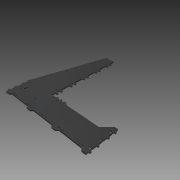
# Autodesk Inventor part: brace_right
Saved by Autodesk Inventor 2014 (Build 180170000, 170)
## iProperties
Created: 2013-12-03
Part Number: brace_right
Material: Generic
Document SubType Name: Modeling
Designer: buben
Density: 1 g/cm^3
Appearance: Anodized - Dark Gray
Author: buben
Subject: Laser Cutted
Autodesk Inventor part; units mm, degrees
ref_plane "YZ Plane" through (0, 0, 0) normal (1, 0, 0) x (0, 1, 0)
ref_plane "XZ Plane" through (0, 0, 0) normal (0, 1, 0) x (-1, 0, 0)
ref_plane "XY Plane" through (0, 0, 0) normal (0, 0, 1) x (1, 0, 0)
sketch "Sketch1" plane through (0, 0, 0) normal (0, 0, 1) x (1, 0, 0)
  line L0 (0, 0) -> (489, 0)
  line L1 (489, 0) -> (489, 150)
  line L2 (0, 0) -> (0, 120)
  line L3 (0, 120) -> (106.25, 518.5)
  line L4 (106.25, 518.5) -> (156.25, 518.5)
  line L5 (156.25, 518.5) -> (156.25, 113.5)
  line L6 (489, 150) -> (474, 150)
  line L7 (474, 150) -> (434, 110)
  line L8 (434, 110) -> (253.25, 110)
  line L9 (253.25, 110) -> (243.25, 120)
  line L10 (243.25, 120) -> (233.25, 120)
  line L11 (233.25, 120) -> (233.25, 113.5)
  line L12 (233.25, 113.5) -> (156.25, 113.5)
  point P0 (244.5, 0)
  dimension "d0" = 489
  dimension "d2" = 120
  dimension "d3" = 45
  dimension "d5" = 6.5
  dimension "d6" = 77
  dimension "d7" = 15
  dimension "d8" = 10
  dimension "d9" = 50
  dimension "d10" = 518.5
  dimension "d13" = 10
  dimension "d261" = 156.25
  dimension "d289" = 150
  dimension "d290" = 40
  constraints: 26 end point, 7 perpendicular, 3 parallel, 1 horizontal, 1 midpoint
  measures "d0" distance of L0.start L0.end
  measures "d2" distance of L0.start L2.end
  measures "d3" angle of L6 L7
  measures "d5" distance of L10.end L11.end
  measures "d6" distance of L11.end L5.end
  measures "d7" distance of L1.end L6.end
  measures "d8" distance of L9.end L10.end
  measures "d9" distance of L3.end L4.end
  measures "d10" distance between parallel lines of L0 L4
  measures "d13" distance between parallel lines of L8 L10
  measures "d261" distance between parallel lines of L2 L5
  measures "d289" distance of L0.end L1.end
  measures "d290" distance between parallel lines of L6 L8
extrude "Extrusion1" add sketch "Sketch1" along normal blind 6.5
sketch "Sketch20" plane through (0, 0, 6.5) normal (0, 0, 1) x (1, 0, 0)
  line L0 (0, 0) -> (489, 0) projected
  line L1 (0, 120) -> (0, 0) projected
  line L2 (16.3, 20.75) -> (16.3, 16.25)
  line L3 (0, 16.25) -> (0, 20.75)
  line L4 (5, 23.25) -> (12.3, 23.25)
  line L5 (12.3, 13.75) -> (5, 13.75)
  line L6 (0, 20.75) -> (5, 20.75)
  line L7 (12.3, 20.75) -> (16.3, 20.75)
  line L8 (16.3, 16.25) -> (12.3, 16.25)
  line L9 (5, 16.25) -> (0, 16.25)
  line L10 (5, 13.75) -> (5, 16.25)
  line L11 (5, 20.75) -> (5, 23.25)
  line L12 (12.3, 23.25) -> (12.3, 20.75)
  line L13 (12.3, 16.25) -> (12.3, 13.75)
  line L14 (16.3, 59.75) -> (16.3, 55.25)
  line L15 (0, 55.25) -> (0, 59.75)
  line L16 (5, 62.25) -> (12.3, 62.25)
  line L17 (12.3, 52.75) -> (5, 52.75)
  line L18 (0, 59.75) -> (5, 59.75)
  line L19 (12.3, 59.75) -> (16.3, 59.75)
  line L20 (16.3, 55.25) -> (12.3, 55.25)
  line L21 (5, 55.25) -> (0, 55.25)
  line L22 (5, 52.75) -> (5, 55.25)
  line L23 (5, 59.75) -> (5, 62.25)
  line L24 (12.3, 62.25) -> (12.3, 59.75)
  line L25 (12.3, 55.25) -> (12.3, 52.75)
  line L26 (16.3, 98.75) -> (16.3, 94.25)
  line L27 (0, 94.25) -> (0, 98.75)
  line L28 (5, 101.25) -> (12.3, 101.25)
  line L29 (12.3, 91.75) -> (5, 91.75)
  line L30 (0, 98.75) -> (5, 98.75)
  line L31 (12.3, 98.75) -> (16.3, 98.75)
  line L32 (16.3, 94.25) -> (12.3, 94.25)
  line L33 (5, 94.25) -> (0, 94.25)
  line L34 (5, 91.75) -> (5, 94.25)
  line L35 (5, 98.75) -> (5, 101.25)
  line L36 (12.3, 101.25) -> (12.3, 98.75)
  line L37 (12.3, 94.25) -> (12.3, 91.75)
  point P0 (16.3, 18.5)
  point P1 (16.3, 57.5)
  point P2 (16.3, 96.5)
  dimension "d291" = 4.5
  dimension "d292" = 5
  dimension "d293" = 4
  dimension "d294" = 7.3
  dimension "d295" = 2.5
  dimension "d296" = 18.5
  dimension "d299" = 39
  constraints: 72 end point, 10 parallel, 6 collinear, 4 perpendicular, 3 horizontal, 1 midpoint, 1 vertical, 50 other
  measures "d291" distance of L2.start L2.end
  measures "d292" distance of L9.start L3.start
  measures "d293" distance of L2.end L8.end
  measures "d294" distance of L5.start L5.end
  measures "d295" distance of L5.end L9.start
  measures "d296" distance from line of L0 point (16.3, 18.5)
  measures "d299" distance of L2.start L19.end
extrude "Extrusion21" cut sketch "Sketch20" against normal through all
sketch "Sketch21" plane through (0, 0, 6.5) normal (0, 0, 1) x (1, 0, 0)
  line L0 (0, 55.25) -> (0, 20.75) projected
  line L1 (16.3, 20.75) -> (16.3, 16.25) projected
  line L2 (0, 16.25) -> (0, 0) projected
  line L3 (0, 120) -> (0, 98.75) projected
  line L4 (16.3, 98.75) -> (16.3, 94.25) projected
  line L5 (0, 94.25) -> (0, 59.75) projected
  line L6 (0, 112) -> (-4.5, 112)
  line L7 (-6.5, 110) -> (-6.5, 106)
  line L8 (-4.5, 104) -> (0, 104)
  line L9 (0, 104) -> (0, 112)
  line L10 (0, 81) -> (-4.5, 81)
  line L11 (-6.5, 79) -> (-6.5, 75)
  line L12 (-4.5, 73) -> (0, 73)
  line L13 (0, 73) -> (0, 81)
  line L14 (0, 42) -> (-4.5, 42)
  line L15 (-6.5, 40) -> (-6.5, 36)
  line L16 (-4.5, 34) -> (0, 34)
  line L17 (0, 34) -> (0, 42)
  line L18 (0, 11) -> (-4.5, 11)
  line L19 (-6.5, 9) -> (-6.5, 5)
  line L20 (-4.5, 3) -> (0, 3)
  line L21 (0, 3) -> (0, 11)
  arc A0 (-6.5, 5) -> (-4.5, 3) centre (-4.5, 5) ccw
  arc A1 (-4.5, 11) -> (-6.5, 9) centre (-4.5, 9) ccw
  arc A2 (-6.5, 36) -> (-4.5, 34) centre (-4.5, 36) ccw
  arc A3 (-4.5, 42) -> (-6.5, 40) centre (-4.5, 40) ccw
  arc A4 (-6.5, 75) -> (-4.5, 73) centre (-4.5, 75) ccw
  arc A5 (-4.5, 81) -> (-6.5, 79) centre (-4.5, 79) ccw
  arc A6 (-6.5, 106) -> (-4.5, 104) centre (-4.5, 106) ccw
  arc A7 (-4.5, 112) -> (-6.5, 110) centre (-4.5, 110) ccw
  point P0 (16.3, 96.5)
  point P1 (16.3, 18.5)
  point P2 (-6.5, 38)
  point P3 (0, 38)
  point P4 (-6.5, 77)
  point P5 (0, 77)
  dimension "d306" = 2
  dimension "d307" = 8
  dimension "d308" = 8
  dimension "d309" = 8
  dimension "d310" = 8
  dimension "d311" = 6.5
  dimension "d312" = 7.5
  dimension "d313" = 7.5
  constraints: 32 end point, 16 point on circle, 16 tangent, 8 centre point, 8 parallel, 7 equal radius, 6 midpoint, 4 horizontal, 4 perpendicular, 4 point on line, 3 collinear, 2 horizontal alignment
  measures "d306" radius of A0
  measures "d307" distance between parallel lines of L20 L18
  measures "d308" distance between parallel lines of L14 L16
  measures "d309" distance between parallel lines of L10 L12
  measures "d310" distance between parallel lines of L6 L8
  measures "d311" distance between parallel lines of L2 L19
  measures "d312" distance from line of L18 point (16.3, 18.5)
  measures "d313" distance from line of L8 point (16.3, 96.5)
extrude "Extrusion22" add sketch "Sketch21" against normal blind 6.5
sketch "Sketch22" plane through (0, 0, 6.5) normal (0, 0, 1) x (1, 0, 0)
  line L0 (233.25, 120) -> (233.25, 113.5) projected
  line L1 (233.25, 113.5) -> (156.25, 113.5) projected
  line L2 (201.5, 113.5) -> (206, 113.5)
  line L3 (206, 97.2) -> (201.5, 97.2)
  line L4 (208.5, 108.5) -> (208.5, 101.2)
  line L5 (199, 101.2) -> (199, 108.5)
  line L6 (206, 113.5) -> (206, 108.5)
  line L7 (206, 101.2) -> (206, 97.2)
  line L8 (201.5, 97.2) -> (201.5, 101.2)
  line L9 (201.5, 108.5) -> (201.5, 113.5)
  line L10 (199, 108.5) -> (201.5, 108.5)
  line L11 (206, 108.5) -> (208.5, 108.5)
  line L12 (208.5, 101.2) -> (206, 101.2)
  line L13 (201.5, 101.2) -> (199, 101.2)
  point P0 (203.75, 97.2)
  dimension "d316" = 4.5
  dimension "d317" = 5
  dimension "d318" = 7.3
  dimension "d319" = 4
  dimension "d320" = 2.5
  dimension "d321" = 29.5
  constraints: 24 end point, 10 parallel, 6 collinear, 4 perpendicular, 3 horizontal, 1 midpoint
  measures "d316" distance of L3.start L3.end
  measures "d317" distance of L2.end L6.end
  measures "d318" distance of L4.start L4.end
  measures "d319" distance of L7.start L3.start
  measures "d320" distance of L8.end L5.start
  measures "d321" distance from line of L0 point (203.75, 97.2)
extrude "Extrusion23" cut sketch "Sketch22" against normal through all
sketch "Sketch23" plane through (0, 0, 6.5) normal (0, 0, 1) x (1, 0, 0)
  line L0 (206, 97.2) -> (201.5, 97.2) projected
  line L1 (201.5, 113.5) -> (156.25, 113.5) projected
  line L2 (243.25, 120) -> (233.25, 120) projected
  line L3 (233.25, 113.5) -> (206, 113.5) projected
  line L4 (196.25, 113.5) -> (188.25, 113.5)
  line L5 (188.25, 113.5) -> (188.25, 118)
  line L6 (190.25, 120) -> (194.25, 120)
  line L7 (196.25, 118) -> (196.25, 113.5)
  line L8 (211.25, 113.5) -> (219.25, 113.5)
  line L9 (219.25, 113.5) -> (219.25, 118)
  line L10 (217.25, 120) -> (213.25, 120)
  line L11 (211.25, 118) -> (211.25, 113.5)
  arc A0 (190.25, 120) -> (188.25, 118) centre (190.25, 118) ccw
  arc A1 (196.25, 118) -> (194.25, 120) centre (194.25, 118) ccw
  arc A2 (213.25, 120) -> (211.25, 118) centre (213.25, 118) ccw
  arc A3 (219.25, 118) -> (217.25, 120) centre (217.25, 118) ccw
  point P0 (203.75, 97.2)
  dimension "d324" = 2
  dimension "d325" = 8
  dimension "d326" = 8
  dimension "d327" = 15
  dimension "d328" = 7.5
  constraints: 16 end point, 8 point on circle, 8 tangent, 4 centre point, 4 parallel, 3 equal radius, 2 collinear, 2 horizontal, 2 perpendicular, 2 point on line, 1 midpoint
  measures "d324" radius of A0
  measures "d325" distance between parallel lines of L7 L5
  measures "d326" distance between parallel lines of L9 L11
  measures "d327" distance between parallel lines of L11 L7
  measures "d328" distance from line of point (203.75, 97.2) L7
extrude "Extrusion24" add sketch "Sketch23" against normal blind 6.5
sketch "Sketch24" plane through (0, 0, 6.5) normal (0, 0, 1) x (1, 0, 0)
  line L0 (0, 3) -> (0, 0) projected
  line L1 (489, 0) -> (489, 150) projected
  line L2 (30, 9.5) -> (38, 9.5)
  line L3 (38, 9.5) -> (38, 3)
  line L4 (38, 3) -> (30, 3)
  line L5 (30, 3) -> (30, 9.5)
  line L6 (53, 9.5) -> (61, 9.5)
  line L7 (61, 9.5) -> (61, 3)
  line L8 (61, 3) -> (53, 3)
  line L9 (53, 3) -> (53, 9.5)
  circle A0 centre (45.5, 6.25) radius 2.25
  line L10 (129.5, 9.5) -> (137.5, 9.5)
  line L11 (137.5, 9.5) -> (137.5, 3)
  line L12 (137.5, 3) -> (129.5, 3)
  line L13 (129.5, 3) -> (129.5, 9.5)
  line L14 (152.5, 9.5) -> (160.5, 9.5)
  line L15 (160.5, 9.5) -> (160.5, 3)
  line L16 (160.5, 3) -> (152.5, 3)
  line L17 (152.5, 3) -> (152.5, 9.5)
  circle A1 centre (145, 6.25) radius 2.25
  line L18 (229, 9.5) -> (237, 9.5)
  line L19 (237, 9.5) -> (237, 3)
  line L20 (237, 3) -> (229, 3)
  line L21 (229, 3) -> (229, 9.5)
  line L22 (252, 9.5) -> (260, 9.5)
  line L23 (260, 9.5) -> (260, 3)
  line L24 (260, 3) -> (252, 3)
  line L25 (252, 3) -> (252, 9.5)
  circle A2 centre (244.5, 6.25) radius 2.25
  line L26 (328.5, 9.5) -> (336.5, 9.5)
  line L27 (336.5, 9.5) -> (336.5, 3)
  line L28 (336.5, 3) -> (328.5, 3)
  line L29 (328.5, 3) -> (328.5, 9.5)
  line L30 (351.5, 9.5) -> (359.5, 9.5)
  line L31 (359.5, 9.5) -> (359.5, 3)
  line L32 (359.5, 3) -> (351.5, 3)
  line L33 (351.5, 3) -> (351.5, 9.5)
  circle A3 centre (344, 6.25) radius 2.25
  line L34 (428, 9.5) -> (436, 9.5)
  line L35 (436, 9.5) -> (436, 3)
  line L36 (436, 3) -> (428, 3)
  line L37 (428, 3) -> (428, 9.5)
  line L38 (451, 9.5) -> (459, 9.5)
  line L39 (459, 9.5) -> (459, 3)
  line L40 (459, 3) -> (451, 3)
  line L41 (451, 3) -> (451, 9.5)
  circle A4 centre (443.5, 6.25) radius 2.25
  line L42 (61, 6.25) -> (129.5, 6.25) construction
  line L43 (160.5, 6.25) -> (229, 6.25) construction
  line L44 (260, 6.25) -> (328.5, 6.25) construction
  line L45 (359.5, 6.25) -> (428, 6.25) construction
  line L46 (0, 0) -> (489, 0) projected
  point P0 (38, 6.25)
  point P1 (137.5, 6.25)
  point P2 (237, 6.25)
  point P3 (336.5, 6.25)
  point P4 (436, 6.25)
  dimension "d331" = 8
  dimension "d332" = 6.5
  dimension "d333" = 15
  dimension "d334" = 4.5
  dimension "d335" = 7.5
  dimension "d336" = 8
  dimension "d337" = 6.5
  dimension "d338" = 15
  dimension "d339" = 4.5
  dimension "d340" = 7.5
  dimension "d341" = 8
  dimension "d342" = 6.5
  dimension "d343" = 15
  dimension "d344" = 4.5
  dimension "d345" = 7.5
  dimension "d346" = 8
  dimension "d347" = 6.5
  dimension "d348" = 15
  dimension "d349" = 4.5
  dimension "d350" = 7.5
  dimension "d351" = 8
  dimension "d352" = 6.5
  dimension "d353" = 15
  dimension "d354" = 4.5
  dimension "d355" = 7.5
  dimension "d356" = 3
  dimension "d357" = 30
  dimension "d358" = 30
  constraints: 88 end point, 22 collinear, 20 parallel, 13 midpoint, 10 horizontal, 10 perpendicular, 5 centre point, 5 horizontal alignment
  measures "d331" distance of L2.start L2.end
  measures "d332" distance of L4.end L2.start
  measures "d333" distance between parallel lines of L9 L3
  measures "d334" diameter of A0
  measures "d335" distance from line of L3 A0.centre
  measures "d336" distance of L13.end L10.end
  measures "d337" distance of L13.start L13.end
  measures "d338" distance between parallel lines of L17 L11
  measures "d339" diameter of A1
  measures "d340" distance from line of L11 A1.centre
  measures "d341" distance of L21.end L18.end
  measures "d342" distance of L21.start L21.end
  measures "d343" distance between parallel lines of L25 L19
  measures "d344" diameter of A2
  measures "d345" distance from line of L19 A2.centre
  measures "d346" distance of L29.end L26.end
  measures "d347" distance of L29.start L29.end
  measures "d348" distance between parallel lines of L33 L27
  measures "d349" diameter of A3
  measures "d350" distance from line of L27 A3.centre
  measures "d351" distance of L37.end L34.end
  measures "d352" distance of L37.start L37.end
  measures "d353" distance between parallel lines of L41 L35
  measures "d354" diameter of A4
  measures "d355" distance from line of L35 A4.centre
  measures "d356" distance between parallel lines of L46 L4
  measures "d357" distance between parallel lines of L0 L5
  measures "d358" distance between parallel lines of L1 L39
extrude "Extrusion25" cut sketch "Sketch24" against normal through all
sketch "Sketch25" plane through (0, 0, 6.5) normal (0, 0, 1) x (1, 0, 0)
  line L0 (156.25, 113.5) -> (156.25, 518.5) projected
  line L1 (156.25, 518.5) -> (106.25, 518.5) projected
  line L2 (156.25, 470.75) -> (156.25, 466.25)
  line L3 (139.95, 466.25) -> (139.95, 470.75)
  line L4 (143.95, 473.25) -> (151.25, 473.25)
  line L5 (151.25, 463.75) -> (143.95, 463.75)
  line L6 (139.95, 470.75) -> (143.95, 470.75)
  line L7 (151.25, 470.75) -> (156.25, 470.75)
  line L8 (156.25, 466.25) -> (151.25, 466.25)
  line L9 (143.95, 466.25) -> (139.95, 466.25)
  line L10 (143.95, 463.75) -> (143.95, 466.25)
  line L11 (143.95, 470.75) -> (143.95, 473.25)
  line L12 (151.25, 473.25) -> (151.25, 470.75)
  line L13 (151.25, 466.25) -> (151.25, 463.75)
  line L14 (156.25, 390.75) -> (156.25, 386.25)
  line L15 (139.95, 386.25) -> (139.95, 390.75)
  line L16 (143.95, 393.25) -> (151.25, 393.25)
  line L17 (151.25, 383.75) -> (143.95, 383.75)
  line L18 (139.95, 390.75) -> (143.95, 390.75)
  line L19 (151.25, 390.75) -> (156.25, 390.75)
  line L20 (156.25, 386.25) -> (151.25, 386.25)
  line L21 (143.95, 386.25) -> (139.95, 386.25)
  line L22 (143.95, 383.75) -> (143.95, 386.25)
  line L23 (143.95, 390.75) -> (143.95, 393.25)
  line L24 (151.25, 393.25) -> (151.25, 390.75)
  line L25 (151.25, 386.25) -> (151.25, 383.75)
  line L26 (156.25, 310.75) -> (156.25, 306.25)
  line L27 (139.95, 306.25) -> (139.95, 310.75)
  line L28 (143.95, 313.25) -> (151.25, 313.25)
  line L29 (151.25, 303.75) -> (143.95, 303.75)
  line L30 (139.95, 310.75) -> (143.95, 310.75)
  line L31 (151.25, 310.75) -> (156.25, 310.75)
  line L32 (156.25, 306.25) -> (151.25, 306.25)
  line L33 (143.95, 306.25) -> (139.95, 306.25)
  line L34 (143.95, 303.75) -> (143.95, 306.25)
  line L35 (143.95, 310.75) -> (143.95, 313.25)
  line L36 (151.25, 313.25) -> (151.25, 310.75)
  line L37 (151.25, 306.25) -> (151.25, 303.75)
  line L38 (156.25, 230.75) -> (156.25, 226.25)
  line L39 (139.95, 226.25) -> (139.95, 230.75)
  line L40 (143.95, 233.25) -> (151.25, 233.25)
  line L41 (151.25, 223.75) -> (143.95, 223.75)
  line L42 (139.95, 230.75) -> (143.95, 230.75)
  line L43 (151.25, 230.75) -> (156.25, 230.75)
  line L44 (156.25, 226.25) -> (151.25, 226.25)
  line L45 (143.95, 226.25) -> (139.95, 226.25)
  line L46 (143.95, 223.75) -> (143.95, 226.25)
  line L47 (143.95, 230.75) -> (143.95, 233.25)
  line L48 (151.25, 233.25) -> (151.25, 230.75)
  line L49 (151.25, 226.25) -> (151.25, 223.75)
  line L50 (156.25, 150.75) -> (156.25, 146.25)
  line L51 (139.95, 146.25) -> (139.95, 150.75)
  line L52 (143.95, 153.25) -> (151.25, 153.25)
  line L53 (151.25, 143.75) -> (143.95, 143.75)
  line L54 (139.95, 150.75) -> (143.95, 150.75)
  line L55 (151.25, 150.75) -> (156.25, 150.75)
  line L56 (156.25, 146.25) -> (151.25, 146.25)
  line L57 (143.95, 146.25) -> (139.95, 146.25)
  line L58 (143.95, 143.75) -> (143.95, 146.25)
  line L59 (143.95, 150.75) -> (143.95, 153.25)
  line L60 (151.25, 153.25) -> (151.25, 150.75)
  line L61 (151.25, 146.25) -> (151.25, 143.75)
  point P0 (139.95, 468.5)
  point P1 (139.95, 388.5)
  point P2 (139.95, 308.5)
  point P3 (139.95, 228.5)
  point P4 (139.95, 148.5)
  dimension "d361" = 4.5
  dimension "d362" = 5
  dimension "d363" = 4
  dimension "d364" = 7.3
  dimension "d365" = 2.5
  dimension "d366" = 50
  dimension "d369" = 80
  constraints: 120 end point, 10 parallel, 6 collinear, 4 perpendicular, 3 horizontal, 1 midpoint, 1 vertical, 100 other
  measures "d361" distance of L3.start L3.end
  measures "d362" distance of L7.start L2.start
  measures "d363" distance of L3.end L6.end
  measures "d364" distance of L4.start L4.end
  measures "d365" distance of L6.end L4.start
  measures "d366" distance from line of L1 point (139.95, 468.5)
  measures "d369" distance of L4.end L16.end
extrude "Extrusion26" cut sketch "Sketch25" against normal through all
sketch "Sketch26" plane through (0, 0, 6.5) normal (0, 0, 1) x (1, 0, 0)
  line L0 (156.25, 390.75) -> (156.25, 466.25) projected
  line L1 (139.95, 466.25) -> (139.95, 470.75) projected
  line L2 (156.25, 470.75) -> (156.25, 518.5) projected
  line L3 (156.25, 484) -> (167.25, 484)
  line L4 (169.25, 482) -> (169.25, 478)
  line L5 (167.25, 476) -> (156.25, 476)
  line L6 (156.25, 476) -> (156.25, 484)
  line L7 (156.25, 461) -> (167.25, 461)
  line L8 (169.25, 459) -> (169.25, 455)
  line L9 (167.25, 453) -> (156.25, 453)
  line L10 (156.25, 453) -> (156.25, 461)
  arc A0 (169.25, 482) -> (167.25, 484) centre (167.25, 482) ccw
  arc A1 (167.25, 476) -> (169.25, 478) centre (167.25, 478) ccw
  arc A2 (169.25, 459) -> (167.25, 461) centre (167.25, 459) ccw
  arc A3 (167.25, 453) -> (169.25, 455) centre (167.25, 455) ccw
  line L11 (156.25, 404) -> (167.25, 404)
  line L12 (169.25, 402) -> (169.25, 398)
  line L13 (167.25, 396) -> (156.25, 396)
  line L14 (156.25, 396) -> (156.25, 404)
  line L15 (156.25, 381) -> (167.25, 381)
  line L16 (169.25, 379) -> (169.25, 375)
  line L17 (167.25, 373) -> (156.25, 373)
  line L18 (156.25, 373) -> (156.25, 381)
  arc A4 (169.25, 402) -> (167.25, 404) centre (167.25, 402) ccw
  arc A5 (167.25, 396) -> (169.25, 398) centre (167.25, 398) ccw
  arc A6 (169.25, 379) -> (167.25, 381) centre (167.25, 379) ccw
  arc A7 (167.25, 373) -> (169.25, 375) centre (167.25, 375) ccw
  line L19 (156.25, 324) -> (167.25, 324)
  line L20 (169.25, 322) -> (169.25, 318)
  line L21 (167.25, 316) -> (156.25, 316)
  line L22 (156.25, 316) -> (156.25, 324)
  line L23 (156.25, 301) -> (167.25, 301)
  line L24 (169.25, 299) -> (169.25, 295)
  line L25 (167.25, 293) -> (156.25, 293)
  line L26 (156.25, 293) -> (156.25, 301)
  arc A8 (169.25, 322) -> (167.25, 324) centre (167.25, 322) ccw
  arc A9 (167.25, 316) -> (169.25, 318) centre (167.25, 318) ccw
  arc A10 (169.25, 299) -> (167.25, 301) centre (167.25, 299) ccw
  arc A11 (167.25, 293) -> (169.25, 295) centre (167.25, 295) ccw
  line L27 (156.25, 244) -> (167.25, 244)
  line L28 (169.25, 242) -> (169.25, 238)
  line L29 (167.25, 236) -> (156.25, 236)
  line L30 (156.25, 236) -> (156.25, 244)
  line L31 (156.25, 221) -> (167.25, 221)
  line L32 (169.25, 219) -> (169.25, 215)
  line L33 (167.25, 213) -> (156.25, 213)
  line L34 (156.25, 213) -> (156.25, 221)
  arc A12 (169.25, 242) -> (167.25, 244) centre (167.25, 242) ccw
  arc A13 (167.25, 236) -> (169.25, 238) centre (167.25, 238) ccw
  arc A14 (169.25, 219) -> (167.25, 221) centre (167.25, 219) ccw
  arc A15 (167.25, 213) -> (169.25, 215) centre (167.25, 215) ccw
  line L35 (156.25, 164) -> (167.25, 164)
  line L36 (169.25, 162) -> (169.25, 158)
  line L37 (167.25, 156) -> (156.25, 156)
  line L38 (156.25, 156) -> (156.25, 164)
  line L39 (156.25, 141) -> (167.25, 141)
  line L40 (169.25, 139) -> (169.25, 135)
  line L41 (167.25, 133) -> (156.25, 133)
  line L42 (156.25, 133) -> (156.25, 141)
  arc A16 (169.25, 162) -> (167.25, 164) centre (167.25, 162) ccw
  arc A17 (167.25, 156) -> (169.25, 158) centre (167.25, 158) ccw
  arc A18 (169.25, 139) -> (167.25, 141) centre (167.25, 139) ccw
  arc A19 (167.25, 133) -> (169.25, 135) centre (167.25, 135) ccw
  point P0 (139.95, 468.5)
  dimension "d376" = 2
  dimension "d377" = 8
  dimension "d378" = 8
  dimension "d379" = 15
  dimension "d380" = 7.5
  dimension "d381" = 13
  dimension "d384" = 80
  constraints: 80 end point, 40 point on circle, 20 centre point, 8 tangent, 4 parallel, 3 equal radius, 2 horizontal, 2 perpendicular, 2 point on line, 1 collinear, 1 midpoint, 1 vertical, 112 other
  measures "d376" radius of A0
  measures "d377" distance between parallel lines of L3 L5
  measures "d378" distance between parallel lines of L9 L7
  measures "d379" distance between parallel lines of L7 L5
  measures "d380" distance from line of point (139.95, 468.5) L5
  measures "d381" distance between parallel lines of L2 L4
  measures "d384" distance of L5.start L13.start
extrude "Extrusion27" add sketch "Sketch26" against normal blind 6.5
sketch "Sketch27" plane through (0, 0, 6.5) normal (0, 0, 1) x (1, 0, 0)
  line L0 (156.25, 518.5) -> (112.25, 518.5)
  line L1 (112.25, 518.5) -> (112.25, 512)
  line L2 (112.25, 512) -> (156.25, 512)
  line L3 (156.25, 512) -> (156.25, 518.5)
  point P0 (106.25, 518.5)
  dimension "d391" = 6.5
  dimension "d392" = 6
  constraints: 8 end point, 2 parallel, 1 horizontal, 1 perpendicular
  measures "d391" distance of L0.end L1.end
  measures "d392" distance from line of point (106.25, 518.5) L1
extrude "Extrusion28" cut sketch "Sketch27" against normal through all
sketch "Sketch28" plane through (0, 0, 6.5) normal (0, 0, 1) x (1, 0, 0)
  line L0 (106.25, 518.5) -> (0, 120) projected
  line L1 (107.1853, 510.363) -> (113.4659, 508.6884) construction
  line L2 (113.4659, 508.6884) -> (9.3854, 118.3254) construction
  line L3 (9.3854, 118.3254) -> (3.1048, 120) construction
  line L4 (3.1048, 120) -> (107.1853, 510.363) construction
  circle A0 centre (27.0612, 197.2353) radius 2.25
  circle A1 centre (47.8773, 275.3079) radius 2.25
  circle A2 centre (68.6934, 353.3805) radius 2.25
  circle A3 centre (89.5095, 431.4531) radius 2.25
  line L5 (6.2451, 119.1627) -> (27.0612, 197.2353) construction
  line L6 (27.0612, 197.2353) -> (47.8773, 275.3079) construction
  line L7 (47.8773, 275.3079) -> (68.6934, 353.3805) construction
  line L8 (68.6934, 353.3805) -> (89.5095, 431.4531) construction
  line L9 (89.5095, 431.4531) -> (110.3256, 509.5257) construction
  line L10 (21.9887, 190.8258) -> (28.2693, 189.1512)
  line L11 (28.2693, 189.1512) -> (26.2083, 181.4212)
  line L12 (26.2083, 181.4212) -> (19.9277, 183.0958)
  line L13 (19.9277, 183.0958) -> (21.9887, 190.8258)
  line L14 (34.1947, 211.3748) -> (32.1337, 203.6449)
  line L15 (27.9141, 213.0494) -> (34.1947, 211.3748)
  line L16 (25.8531, 205.3194) -> (27.9141, 213.0494)
  line L17 (32.1337, 203.6449) -> (25.8531, 205.3194)
  line L18 (55.0108, 289.4474) -> (52.9498, 281.7175)
  line L19 (48.7302, 291.122) -> (55.0108, 289.4474)
  line L20 (46.6692, 283.392) -> (48.7302, 291.122)
  line L21 (52.9498, 281.7175) -> (46.6692, 283.392)
  line L22 (49.0854, 267.2238) -> (47.0244, 259.4938)
  line L23 (42.8048, 268.8984) -> (49.0854, 267.2238)
  line L24 (40.7438, 261.1684) -> (42.8048, 268.8984)
  line L25 (47.0244, 259.4938) -> (40.7438, 261.1684)
  line L26 (75.8269, 367.52) -> (73.7659, 359.7901)
  line L27 (69.5463, 369.1946) -> (75.8269, 367.52)
  line L28 (67.4853, 361.4646) -> (69.5463, 369.1946)
  line L29 (73.7659, 359.7901) -> (67.4853, 361.4646)
  line L30 (69.9015, 345.2964) -> (67.8405, 337.5664)
  line L31 (63.6209, 346.971) -> (69.9015, 345.2964)
  line L32 (61.5599, 339.241) -> (63.6209, 346.971)
  line L33 (67.8405, 337.5664) -> (61.5599, 339.241)
  line L34 (96.643, 445.5926) -> (94.582, 437.8627)
  line L35 (90.3624, 447.2672) -> (96.643, 445.5926)
  line L36 (88.3014, 439.5372) -> (90.3624, 447.2672)
  line L37 (94.582, 437.8627) -> (88.3014, 439.5372)
  line L38 (90.7176, 423.369) -> (88.6566, 415.639)
  line L39 (84.437, 425.0435) -> (90.7176, 423.369)
  line L40 (82.376, 417.3136) -> (84.437, 425.0435)
  line L41 (88.6566, 415.639) -> (82.376, 417.3136)
  dimension "d395" = 6.5
  dimension "d396" = 3.25
  dimension "d397" = 3.25
  dimension "d398" = 3.25
  dimension "d399" = 3.25
  dimension "d400" = 4.5
  dimension "d401" = 404
  dimension "d402" = 8
  dimension "d403" = 15
  dimension "d404" = 15
  dimension "d405" = 15
  dimension "d406" = 15
  dimension "d407" = 7.5
  dimension "d408" = 7.5
  dimension "d409" = 7.5
  dimension "d410" = 7.5
  dimension "d411" = 3
  constraints: 82 end point, 19 parallel, 17 collinear, 11 equal length, 9 perpendicular, 4 centre point, 3 equal radius, 2 midpoint, 1 horizontal alignment
  measures "d395" distance between parallel lines of L4 L2
  measures "d396" distance from line of L2 L6.start
  measures "d397" distance from line of L2 L6.end
  measures "d398" distance from line of L2 L7.end
  measures "d399" distance from line of L2 L9.start
  measures "d400" diameter of A0
  measures "d401" distance of L2.start L2.end
  measures "d402" distance of L12.end L13.end
  measures "d403" distance between parallel lines of L17 L10
  measures "d404" distance between parallel lines of L21 L23
  measures "d405" distance between parallel lines of L29 L31
  measures "d406" distance between parallel lines of L37 L39
  measures "d407" distance from line of L6.start L10
  measures "d408" distance from line of L6.end L23
  measures "d409" distance from line of L7.end L31
  measures "d410" distance from line of L9.start L39
  measures "d411" distance between parallel lines of L0 L4
extrude "Extrusion29" cut sketch "Sketch28" against normal through all
sketch "Sketch29" plane through (0, 0, 6.5) normal (0, 0, 1) x (1, 0, 0)
  line L0 (156.25, 484) -> (156.25, 512) projected
  line L1 (156.25, 512) -> (112.25, 512) projected
  line L2 (126, 512) -> (130.5, 512)
  line L3 (130.5, 495.7) -> (126, 495.7)
  line L4 (133, 507) -> (133, 499.7)
  line L5 (123.5, 499.7) -> (123.5, 507)
  line L6 (133, 499.7) -> (130.5, 499.7)
  line L7 (126, 499.7) -> (123.5, 499.7)
  line L8 (123.5, 507) -> (126, 507)
  line L9 (130.5, 507) -> (133, 507)
  line L10 (126, 495.7) -> (126, 499.7)
  line L11 (126, 507) -> (126, 512)
  line L12 (130.5, 512) -> (130.5, 507)
  line L13 (130.5, 499.7) -> (130.5, 495.7)
  point P0 (128.25, 495.7)
  dimension "d414" = 4.5
  dimension "d415" = 5
  dimension "d416" = 7.3
  dimension "d417" = 4
  dimension "d418" = 2.5
  dimension "d419" = 28
  constraints: 24 end point, 10 parallel, 6 collinear, 4 perpendicular, 3 horizontal, 1 midpoint
  measures "d414" distance of L3.start L3.end
  measures "d415" distance of L8.end L2.start
  measures "d416" distance of L5.start L5.end
  measures "d417" distance of L3.end L7.start
  measures "d418" distance of L7.start L5.start
  measures "d419" distance from line of L0 point (128.25, 495.7)
extrude "Extrusion30" cut sketch "Sketch29" against normal through all
sketch "Sketch30" plane through (0, 0, 6.5) normal (0, 0, 1) x (1, 0, 0)
  line L0 (112.25, 518.5) -> (106.25, 518.5) projected
  line L1 (156.25, 404) -> (156.25, 453) projected
  line L2 (113.25, 451) -> (121.25, 451)
  line L3 (121.25, 451) -> (121.25, 444.5)
  line L4 (121.25, 444.5) -> (113.25, 444.5)
  line L5 (113.25, 444.5) -> (113.25, 451)
  circle A0 centre (128.75, 447.75) radius 2.25
  point P0 (121.25, 447.75)
  dimension "d422" = 6.5
  dimension "d423" = 8
  dimension "d424" = 4.5
  dimension "d425" = 7.5
  dimension "d426" = 27.5
  dimension "d427" = 74
  constraints: 8 end point, 2 parallel, 1 centre point, 1 horizontal, 1 horizontal alignment, 1 midpoint, 1 perpendicular
  measures "d422" distance of L4.end L2.start
  measures "d423" distance of L2.start L2.end
  measures "d424" diameter of A0
  measures "d425" distance from line of L3 A0.centre
  measures "d426" distance from line of L1 A0.centre
  measures "d427" distance between parallel lines of L0 L4
extrude "Extrusion31" cut sketch "Sketch30" against normal through all
sketch "Sketch31" plane through (0, 0, 6.5) normal (0, 0, 1) x (1, 0, 0)
  line L0 (0, 0) -> (489, 0) projected
  line L1 (489, 0) -> (489, 150) projected
  line L2 (489, 20.75) -> (489, 16.25)
  line L3 (472.7, 16.25) -> (472.7, 20.75)
  line L4 (476.7, 23.25) -> (484, 23.25)
  line L5 (484, 13.75) -> (476.7, 13.75)
  line L6 (472.7, 20.75) -> (476.7, 20.75)
  line L7 (484, 20.75) -> (489, 20.75)
  line L8 (489, 16.25) -> (484, 16.25)
  line L9 (476.7, 16.25) -> (472.7, 16.25)
  line L10 (476.7, 13.75) -> (476.7, 16.25)
  line L11 (476.7, 20.75) -> (476.7, 23.25)
  line L12 (484, 23.25) -> (484, 20.75)
  line L13 (484, 16.25) -> (484, 13.75)
  line L14 (489, 72.75) -> (489, 68.25)
  line L15 (472.7, 68.25) -> (472.7, 72.75)
  line L16 (476.7, 75.25) -> (484, 75.25)
  line L17 (484, 65.75) -> (476.7, 65.75)
  line L18 (472.7, 72.75) -> (476.7, 72.75)
  line L19 (484, 72.75) -> (489, 72.75)
  line L20 (489, 68.25) -> (484, 68.25)
  line L21 (476.7, 68.25) -> (472.7, 68.25)
  line L22 (476.7, 65.75) -> (476.7, 68.25)
  line L23 (476.7, 72.75) -> (476.7, 75.25)
  line L24 (484, 75.25) -> (484, 72.75)
  line L25 (484, 68.25) -> (484, 65.75)
  line L26 (489, 124.75) -> (489, 120.25)
  line L27 (472.7, 120.25) -> (472.7, 124.75)
  line L28 (476.7, 127.25) -> (484, 127.25)
  line L29 (484, 117.75) -> (476.7, 117.75)
  line L30 (472.7, 124.75) -> (476.7, 124.75)
  line L31 (484, 124.75) -> (489, 124.75)
  line L32 (489, 120.25) -> (484, 120.25)
  line L33 (476.7, 120.25) -> (472.7, 120.25)
  line L34 (476.7, 117.75) -> (476.7, 120.25)
  line L35 (476.7, 124.75) -> (476.7, 127.25)
  line L36 (484, 127.25) -> (484, 124.75)
  line L37 (484, 120.25) -> (484, 117.75)
  line L38 (472.7, 18.5) -> (472.7, 70.5) construction
  line L39 (472.7, 70.5) -> (472.7, 122.5) construction
  dimension "d430" = 4.5
  dimension "d431" = 5
  dimension "d432" = 7.3
  dimension "d433" = 4
  dimension "d434" = 2.5
  dimension "d435" = 4.5
  dimension "d436" = 5
  dimension "d437" = 7.3
  dimension "d438" = 4
  dimension "d439" = 2.5
  dimension "d440" = 4.5
  dimension "d441" = 5
  dimension "d442" = 7.3
  dimension "d443" = 4
  dimension "d444" = 2.5
  dimension "d445" = 18.5
  dimension "d446" = 52
  constraints: 76 end point, 30 parallel, 19 collinear, 12 perpendicular, 9 horizontal, 3 midpoint
  measures "d430" distance of L3.start L3.end
  measures "d431" distance of L7.start L2.start
  measures "d432" distance of L4.start L4.end
  measures "d433" distance of L3.end L6.end
  measures "d434" distance of L6.end L4.start
  measures "d435" distance of L15.start L18.start
  measures "d436" distance of L24.end L19.end
  measures "d437" distance of L16.start L16.end
  measures "d438" distance of L18.start L23.start
  measures "d439" distance of L23.start L16.start
  measures "d440" distance of L27.start L30.start
  measures "d441" distance of L36.end L31.end
  measures "d442" distance of L28.start L28.end
  measures "d443" distance of L30.start L35.start
  measures "d444" distance of L35.start L28.start
  measures "d445" distance from line of L0 L38.start
  measures "d446" distance of L38.start L38.end
extrude "Extrusion32" cut sketch "Sketch31" against normal through all
sketch "Sketch32" plane through (0, 0, 6.5) normal (0, 0, 1) x (1, 0, 0)
  line L0 (489, 72.75) -> (489, 120.25) projected
  line L1 (472.7, 120.25) -> (472.7, 124.75) projected
  line L2 (489, 124.75) -> (489, 150) projected
  line L3 (489, 0) -> (489, 16.25) projected
  line L4 (472.7, 16.25) -> (472.7, 20.75) projected
  line L5 (489, 20.75) -> (489, 68.25) projected
  line L6 (489, 11) -> (493.5, 11)
  line L7 (495.5, 9) -> (495.5, 5)
  line L8 (493.5, 3) -> (489, 3)
  line L9 (489, 3) -> (489, 11)
  line L10 (489, 48.5) -> (493.5, 48.5)
  line L11 (495.5, 46.5) -> (495.5, 42.5)
  line L12 (493.5, 40.5) -> (489, 40.5)
  line L13 (489, 40.5) -> (489, 48.5)
  line L14 (489, 100.5) -> (493.5, 100.5)
  line L15 (495.5, 98.5) -> (495.5, 94.5)
  line L16 (493.5, 92.5) -> (489, 92.5)
  line L17 (489, 92.5) -> (489, 100.5)
  line L18 (489, 138) -> (493.5, 138)
  line L19 (495.5, 136) -> (495.5, 132)
  line L20 (493.5, 130) -> (489, 130)
  line L21 (489, 130) -> (489, 138)
  arc A0 (495.5, 136) -> (493.5, 138) centre (493.5, 136) ccw
  arc A1 (493.5, 130) -> (495.5, 132) centre (493.5, 132) ccw
  arc A2 (495.5, 98.5) -> (493.5, 100.5) centre (493.5, 98.5) ccw
  arc A3 (493.5, 92.5) -> (495.5, 94.5) centre (493.5, 94.5) ccw
  arc A4 (495.5, 46.5) -> (493.5, 48.5) centre (493.5, 46.5) ccw
  arc A5 (493.5, 40.5) -> (495.5, 42.5) centre (493.5, 42.5) ccw
  arc A6 (495.5, 9) -> (493.5, 11) centre (493.5, 9) ccw
  arc A7 (493.5, 3) -> (495.5, 5) centre (493.5, 5) ccw
  point P0 (495.5, 96.5)
  point P1 (489, 96.5)
  point P2 (495.5, 44.5)
  point P3 (489, 44.5)
  point P4 (472.7, 18.5)
  point P5 (472.7, 122.5)
  dimension "d449" = 2
  dimension "d450" = 8
  dimension "d451" = 8
  dimension "d452" = 8
  dimension "d453" = 8
  dimension "d454" = 6.5
  dimension "d455" = 7.5
  dimension "d456" = 7.5
  constraints: 32 end point, 16 point on circle, 16 tangent, 8 centre point, 8 parallel, 7 equal radius, 6 midpoint, 4 horizontal, 4 perpendicular, 4 point on line, 3 collinear, 2 horizontal alignment
  measures "d449" radius of A0
  measures "d450" distance between parallel lines of L8 L6
  measures "d451" distance between parallel lines of L10 L12
  measures "d452" distance between parallel lines of L16 L14
  measures "d453" distance between parallel lines of L20 L18
  measures "d454" distance between parallel lines of L3 L7
  measures "d455" distance from line of L20 point (472.7, 122.5)
  measures "d456" distance from line of L6 point (472.7, 18.5)
extrude "Extrusion33" add sketch "Sketch32" against normal blind 6.5
sketch "Sketch33" plane through (0, 0, 6.5) normal (0, 0, 1) x (1, 0, 0)
  line L0 (0, 0) -> (489, 0) projected
  line L1 (489, 48.5) -> (489, 68.25) projected
  line L2 (0, 0) -> (0, -10)
  line L3 (0, -10) -> (20, -10)
  line L4 (20, -10) -> (30, 0)
  line L5 (0, 0) -> (30, 0)
  line L6 (146.3333, 0) -> (156.3333, -10)
  line L7 (156.3333, -10) -> (176.3333, -10)
  line L8 (176.3333, -10) -> (186.3333, 0)
  line L9 (186.3333, 0) -> (146.3333, 0)
  line L10 (302.6667, 0) -> (312.6667, -10)
  line L11 (312.6667, -10) -> (332.6667, -10)
  line L12 (332.6667, -10) -> (342.6667, 0)
  line L13 (302.6667, 0) -> (342.6667, 0)
  line L14 (489, 0) -> (489, -10)
  line L15 (489, -10) -> (469, -10)
  line L16 (469, -10) -> (459, 0)
  line L17 (489, 0) -> (459, 0)
  line L18 (20, -10) -> (156.3333, -10) construction
  line L19 (176.3333, -10) -> (312.6667, -10) construction
  line L20 (332.6667, -10) -> (469, -10) construction
  dimension "d459" = 45
  dimension "d460" = 10
  dimension "d461" = 20
  constraints: 38 end point, 14 collinear, 8 perpendicular, 6 point on line, 3 parallel
  measures "d459" angle of L5 L4
  measures "d460" distance of L0.start L2.end
  measures "d461" distance of L2.end L3.end
extrude "Extrusion34" add sketch "Sketch33" against normal blind 6.5
sketch "Sketch34" plane through (0, 0, 6.5) normal (0, 0, 1) x (1, 0, 0)
  line L0 (0, 34) -> (0, 20.75) projected
  line L1 (20, 51) -> (28, 51)
  line L2 (28, 51) -> (28, 44.5)
  line L3 (28, 44.5) -> (20, 44.5)
  line L4 (20, 44.5) -> (20, 51)
  line L5 (128.25, 51) -> (136.25, 51)
  line L6 (136.25, 51) -> (136.25, 44.5)
  line L7 (136.25, 44.5) -> (128.25, 44.5)
  line L8 (128.25, 44.5) -> (128.25, 51)
  circle A0 centre (50, 47.75) radius 2.25
  point P0 (30, 0)
  point P1 (0, 0)
  point P2 (28, 47.75)
  dimension "d464" = 8
  dimension "d465" = 6.5
  dimension "d466" = 4.5
  dimension "d467" = 100.25
  dimension "d468" = 22
  dimension "d469" = 20
  dimension "d470" = 44.5
  constraints: 16 end point, 4 parallel, 3 collinear, 2 horizontal, 2 perpendicular, 1 centre point, 1 horizontal alignment, 1 midpoint
  measures "d464" distance of L1.start L1.end
  measures "d465" distance of L3.end L1.start
  measures "d466" diameter of A0
  measures "d467" distance between parallel lines of L8 L2
  measures "d468" distance from line of A0.centre L2
  measures "d469" distance between parallel lines of L0 L4
  measures "d470" distance from line of point (30, 0) L3
extrude "Extrusion35" cut sketch "Sketch34" against normal through all
sketch "Sketch35" plane through (0, 0, 6.5) normal (0, 0, 1) x (1, 0, 0)
  line L0 (20, 44.5) -> (20, 51) projected
  line L1 (20, 51) -> (28, 51) projected
  line L2 (0, 73) -> (0, 59.75) projected
  line L3 (40, 71) -> (40, 56) construction
  line L4 (36, 71) -> (36, 56)
  line L5 (44, 56) -> (44, 71)
  arc A0 (44, 71) -> (36, 71) centre (40, 71) ccw
  arc A1 (36, 56) -> (44, 56) centre (40, 56) ccw
  point P0 (0, 0)
  point P1 (40, 63.5)
  dimension "d473" = 8
  dimension "d474" = 15
  dimension "d475" = 40
  dimension "d476" = 5
  constraints: 8 end point, 4 point on circle, 4 tangent, 2 centre point, 2 parallel, 1 midpoint
  measures "d473" distance between parallel lines of L5 L4
  measures "d474" distance of L3.start L3.end
  measures "d475" distance between parallel lines of L2 L3
  measures "d476" distance from line of L1 L3.end
extrude "Extrusion36" cut sketch "Sketch35" against normal through all
sketch "Sketch36" plane through (0, 0, 6.5) normal (0, 0, 1) x (1, 0, 0)
  line L0 (489, 138) -> (489, 150) projected
  line L1 (489, 150) -> (474, 150) projected
  line L2 (477, 147) -> (485, 147)
  line L3 (485, 147) -> (485, 140.5)
  line L4 (485, 140.5) -> (477, 140.5)
  line L5 (477, 140.5) -> (477, 147)
  point P0 (0, 0)
  dimension "d479" = 8
  dimension "d480" = 6.5
  dimension "d481" = 4
  dimension "d482" = 3
  constraints: 8 end point, 2 parallel, 1 horizontal, 1 perpendicular
  measures "d479" distance of L3.end L4.end
  measures "d480" distance of L4.end L2.start
  measures "d481" distance between parallel lines of L0 L3
  measures "d482" distance between parallel lines of L2 L1
extrude "Extrusion37" cut sketch "Sketch36" against normal through all
body "Solid1"
